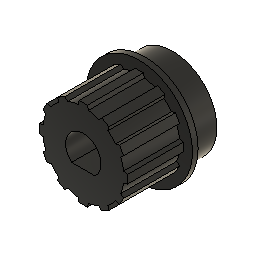
ENGRENAGEM_PEQUENA Modificada v1 (Autodesk Fusion 360 design; units mm, degrees)
Autodesk Fusion 360 part; units mm, degrees
sketch "Esboço1" plane through (0, 0, 0) normal (0, 1, 0) x (1, 0, 0)
  circle A0 centre (0, 0) radius 7.825
  line L0 (7.825, 0) -> (-7.825, 0) construction
  line L1 (0, 0) -> (0, -9.175) construction
  line L2 (0, 0) -> (0, 9.175) construction
  circle A1 centre (0, 0) radius 4
  circle A2 centre (0, 0) radius 9.175
  line L3 (-0.935, -9.9864) -> (0.935, -9.9864)
  line L4 (-1.55, -7.6699) -> (1.55, -7.6699)
  line L5 (-1.55, -7.6699) -> (-0.935, -9.9864)
  line L6 (0.935, -9.9864) -> (1.55, -7.6699)
  line L7 (4.1835, -9.116) -> (5.8029, -8.181)
  line L8 (2.4926, -7.4174) -> (5.1773, -5.8674)
  line L9 (2.4926, -7.4174) -> (4.1835, -9.116)
  line L10 (5.8029, -8.181) -> (5.1773, -5.8674)
  line L11 (8.181, -5.8029) -> (9.116, -4.1835)
  line L12 (5.8674, -5.1773) -> (7.4174, -2.4926)
  line L13 (5.8674, -5.1773) -> (8.181, -5.8029)
  line L14 (9.116, -4.1835) -> (7.4174, -2.4926)
  line L15 (9.9864, -0.935) -> (9.9864, 0.935)
  line L16 (7.6699, -1.55) -> (7.6699, 1.55)
  line L17 (7.6699, -1.55) -> (9.9864, -0.935)
  line L18 (9.9864, 0.935) -> (7.6699, 1.55)
  line L19 (9.116, 4.1835) -> (8.181, 5.8029)
  line L20 (7.4174, 2.4926) -> (5.8674, 5.1773)
  line L21 (7.4174, 2.4926) -> (9.116, 4.1835)
  line L22 (8.181, 5.8029) -> (5.8674, 5.1773)
  line L23 (5.8029, 8.181) -> (4.1835, 9.116)
  line L24 (5.1773, 5.8674) -> (2.4926, 7.4174)
  line L25 (5.1773, 5.8674) -> (5.8029, 8.181)
  line L26 (4.1835, 9.116) -> (2.4926, 7.4174)
  line L27 (0.935, 9.9864) -> (-0.935, 9.9864)
  line L28 (1.55, 7.6699) -> (-1.55, 7.6699)
  line L29 (1.55, 7.6699) -> (0.935, 9.9864)
  line L30 (-0.935, 9.9864) -> (-1.55, 7.6699)
  line L31 (-4.1835, 9.116) -> (-5.8029, 8.181)
  line L32 (-2.4926, 7.4174) -> (-5.1773, 5.8674)
  line L33 (-2.4926, 7.4174) -> (-4.1835, 9.116)
  line L34 (-5.8029, 8.181) -> (-5.1773, 5.8674)
  line L35 (-8.181, 5.8029) -> (-9.116, 4.1835)
  line L36 (-5.8674, 5.1773) -> (-7.4174, 2.4926)
  line L37 (-5.8674, 5.1773) -> (-8.181, 5.8029)
  line L38 (-9.116, 4.1835) -> (-7.4174, 2.4926)
  line L39 (-9.9864, 0.935) -> (-9.9864, -0.935)
  line L40 (-7.6699, 1.55) -> (-7.6699, -1.55)
  line L41 (-7.6699, 1.55) -> (-9.9864, 0.935)
  line L42 (-9.9864, -0.935) -> (-7.6699, -1.55)
  line L43 (-9.116, -4.1835) -> (-8.181, -5.8029)
  line L44 (-7.4174, -2.4926) -> (-5.8674, -5.1773)
  line L45 (-7.4174, -2.4926) -> (-9.116, -4.1835)
  line L46 (-8.181, -5.8029) -> (-5.8674, -5.1773)
  line L47 (-5.8029, -8.181) -> (-4.1835, -9.116)
  line L48 (-5.1773, -5.8674) -> (-2.4926, -7.4174)
  line L49 (-5.1773, -5.8674) -> (-5.8029, -8.181)
  line L50 (-4.1835, -9.116) -> (-2.4926, -7.4174)
  dimension "d1" = 15.65
  dimension "d3" = 9.175
  dimension "d4" = 9.175
  dimension "d10" = 8
  dimension "d33" = 18.35
  dimension "d42" = 1.87
  dimension "d43" = 3.1
  dimension "d47" = 1.55
  dimension "d48" = 0.935
  dimension "d50" = 360
  constraint coincident A0.centre L1.start
  constraint coincident A0 L0.start
  constraint coincident A0 L0.end
  constraint perpendicular L0 L1
  constraint perpendicular L0 L2
  constraint concentric A0 A2
  constraint perpendicular L1 L3
  constraint perpendicular L1 L4
  constraint coincident L1.end A2
  constraint vertical L1
  constraint coincident A0 L4.end
  measures "d1" diameter of A0
  measures "d3" distance of A0.centre L1.end
  measures "d4" distance of A0.centre L2.end
  measures "d10" diameter of A1
  measures "d33" diameter of A2
  measures "d42" distance of L3.start L3.end
  measures "d43" distance of L4.start L4.end
  measures "d47" distance of L1 L4.start
  measures "d48" distance of L1 L3.start
extrude "Extrusão1" add sketch "Esboço1" along normal blind 12.65 makes body 1
sketch "Esboço2" plane through (0, 12.65, 0) normal (0, 1, 0) x (-1, 0, 0)
  circle A0 centre (0, 0) radius 4
  circle A1 centre (0, 0) radius 12
  line L0 (4.1835, 9.116) -> (3.5365, 8.466)
  arc A2 (3.5365, 8.466) -> (1.1703, 9.1001) centre (0, 0) ccw
  line L1 (1.1703, 9.1001) -> (0.935, 9.9864)
  line L2 (0.935, 9.9864) -> (-0.935, 9.9864)
  line L3 (-0.935, 9.9864) -> (-1.1703, 9.1001)
  arc A3 (-1.1703, 9.1001) -> (-3.5365, 8.466) centre (0, 0) ccw
  line L4 (-3.5365, 8.466) -> (-4.1835, 9.116)
  line L5 (-4.1835, 9.116) -> (-5.8029, 8.181)
  line L6 (-5.8029, 8.181) -> (-5.5636, 7.2957)
  arc A4 (-5.5636, 7.2957) -> (-7.2957, 5.5636) centre (0, 0) ccw
  line L7 (-7.2957, 5.5636) -> (-8.181, 5.8029)
  line L8 (-8.181, 5.8029) -> (-9.116, 4.1835)
  line L9 (-9.116, 4.1835) -> (-8.466, 3.5365)
  arc A5 (-8.466, 3.5365) -> (-9.1001, 1.1703) centre (0, 0) ccw
  line L10 (-9.1001, 1.1703) -> (-9.9864, 0.935)
  line L11 (-9.9864, 0.935) -> (-9.9864, -0.935)
  line L12 (-9.9864, -0.935) -> (-9.1001, -1.1703)
  arc A6 (-9.1001, -1.1703) -> (-8.466, -3.5365) centre (0, 0) ccw
  line L13 (-8.466, -3.5365) -> (-9.116, -4.1835)
  line L14 (-9.116, -4.1835) -> (-8.181, -5.8029)
  line L15 (-8.181, -5.8029) -> (-7.2957, -5.5636)
  arc A7 (-7.2957, -5.5636) -> (-5.5636, -7.2957) centre (0, 0) ccw
  line L16 (-5.5636, -7.2957) -> (-5.8029, -8.181)
  line L17 (-5.8029, -8.181) -> (-4.1835, -9.116)
  line L18 (-4.1835, -9.116) -> (-3.5365, -8.466)
  arc A8 (-3.5365, -8.466) -> (-1.1703, -9.1001) centre (0, 0) ccw
  line L19 (-1.1703, -9.1001) -> (-0.935, -9.9864)
  line L20 (-0.935, -9.9864) -> (0.935, -9.9864)
  line L21 (0.935, -9.9864) -> (1.1703, -9.1001)
  arc A9 (1.1703, -9.1001) -> (3.5365, -8.466) centre (0, 0) ccw
  line L22 (3.5365, -8.466) -> (4.1835, -9.116)
  line L23 (4.1835, -9.116) -> (5.8029, -8.181)
  line L24 (5.8029, -8.181) -> (5.5636, -7.2957)
  arc A10 (5.5636, -7.2957) -> (7.2957, -5.5636) centre (0, 0) ccw
  line L25 (7.2957, -5.5636) -> (8.181, -5.8029)
  line L26 (8.181, -5.8029) -> (9.116, -4.1835)
  line L27 (9.116, -4.1835) -> (8.466, -3.5365)
  arc A11 (8.466, -3.5365) -> (9.1001, -1.1703) centre (0, 0) ccw
  line L28 (9.1001, -1.1703) -> (9.9864, -0.935)
  line L29 (9.9864, -0.935) -> (9.9864, 0.935)
  line L30 (9.9864, 0.935) -> (9.1001, 1.1703)
  arc A12 (9.1001, 1.1703) -> (8.466, 3.5365) centre (0, 0) ccw
  line L31 (8.466, 3.5365) -> (9.116, 4.1835)
  line L32 (9.116, 4.1835) -> (8.181, 5.8029)
  line L33 (8.181, 5.8029) -> (7.2957, 5.5636)
  arc A13 (7.2957, 5.5636) -> (5.5636, 7.2957) centre (0, 0) ccw
  line L34 (5.5636, 7.2957) -> (5.8029, 8.181)
  line L35 (5.8029, 8.181) -> (4.1835, 9.116)
  dimension "d13" = 24
  constraint coincident A0.centre A1.centre
  measures "d13" diameter of A1
extrude "Extrusão2" add sketch "Esboço2" along normal blind 1.3 separate body contours A1 | L0 A2 L1 L2 L3 A3 L4 L5 L6 A4 L7 L8 L9 A5 L10 L11 L12 A6 L13 L14 L15 A7 L16 L17 L18 A8 L19 L20 L21 A9 L22 L23 L24 A10 L25 L26 L27 A11 L28 L29 L30 A12 L31 L32 L33 A13 L34 L35 makes body 2
sketch "Esboço3" plane through (0, 13.95, 0) normal (0, 1, 0) x (-1, 0, 0)
  circle A0 centre (0, 0) radius 4
  circle A1 centre (0, 0) radius 12
  circle A2 centre (0, 0) radius 10
  dimension "d16" = 20
  constraint coincident A0.centre A1.centre
  measures "d16" diameter of A2
extrude "Extrusão3" add sketch "Esboço3" along normal blind 6.25 contours A2 bodies 2
sketch "Esboço4" plane through (0, 20.2, 0) normal (0, 1, 0) x (-1, 0, 0)
  circle A0 centre (0, 0) radius 4
  circle A1 centre (0, 0) radius 10
  circle A2 centre (0, 0) radius 6
  line L0 (0, 0) -> (0, -8.9799) construction
  line L1 (0, -5.9921) -> (-2.85, -5.9921)
  line L2 (-2.85, -5.9921) -> (-2.85, -7.9921)
  line L3 (-2.85, -7.9921) -> (0, -7.9921)
  line L4 (0, -5.9921) -> (2.85, -5.9921)
  line L5 (2.85, -5.9921) -> (2.85, -7.9921)
  line L6 (2.85, -7.9921) -> (0, -7.9921)
  line L7 (2.85, -5.9921) -> (2.85, -5.2799)
  line L8 (-2.85, -5.9921) -> (-2.85, -5.2799)
  dimension "d19" = 12
  dimension "d20" = 2.85
  dimension "d21" = 2.85
  dimension "d22" = 2
  constraint coincident A0.centre A1.centre
  constraint vertical L0
  constraint coincident L0 L1.start
  constraint perpendicular L0 L1
  constraint perpendicular L1 L2
  constraint coincident L0 L3.end
  constraint perpendicular L2 L3
  constraint perpendicular L0 L4
  constraint perpendicular L4 L5
  constraint perpendicular L0 L6
  constraint coincident A2 L7.end
  constraint perpendicular L4 L7
  constraint symmetric L0 L4.end L1.end
  constraint symmetric L0 L7.end L8.end
  measures "d19" diameter of A2
  measures "d20" distance of L3.end L5.end
  measures "d21" distance of L2.end L3.end
  measures "d22" distance of L4.end L5.end
extrude "Extrusão4" cut sketch "Esboço4" against normal blind 6 contours A2 L1 L8 | A2 L4 L7 | A2 L1 L2 L3 L4 L5 L6 bodies 2
sketch "Esboço5" plane through (0, 0, -7.9921) normal (0, 0, 1) x (-1, 0, 0)
  line L0 (-2.85, -20.2) -> (2.85, -20.2)
  line L1 (2.85, -20.2) -> (2.85, -14.2)
  line L2 (2.85, -14.2) -> (-2.85, -14.2)
  line L3 (-2.85, -14.2) -> (-2.85, -20.2)
  circle A0 centre (0, -17) radius 1.65
  dimension "d25" = 3.3
  measures "d25" diameter of A0
extrude "Extrusão5" cut sketch "Esboço5" along normal blind 5 and the other way blind 2.008 contours A0 bodies 2
sketch "Esboço6" plane through (0, 0, 0) normal (0, -1, 0) x (1, 0, 0)
  circle A0 centre (0, 0) radius 4
  line L0 (0, -4) -> (0, -3) construction
  line L1 (0, -3) -> (-2.6458, -3)
  line L2 (0, -3) -> (2.6458, -3)
  line L3 (-3.5365, 8.466) -> (-4.1835, 9.116)
  line L4 (-4.1835, 9.116) -> (-5.8029, 8.181)
  line L5 (-5.8029, 8.181) -> (-5.5636, 7.2957)
  arc A1 (-5.5636, 7.2957) -> (-7.2957, 5.5636) centre (0, 0) ccw
  line L6 (-7.2957, 5.5636) -> (-8.181, 5.8029)
  line L7 (-8.181, 5.8029) -> (-9.116, 4.1835)
  line L8 (-9.116, 4.1835) -> (-8.466, 3.5365)
  arc A2 (-8.466, 3.5365) -> (-9.1001, 1.1703) centre (0, 0) ccw
  line L9 (-9.1001, 1.1703) -> (-9.9864, 0.935)
  line L10 (-9.9864, 0.935) -> (-9.9864, -0.935)
  line L11 (-9.9864, -0.935) -> (-9.1001, -1.1703)
  arc A3 (-9.1001, -1.1703) -> (-8.466, -3.5365) centre (0, 0) ccw
  line L12 (-8.466, -3.5365) -> (-9.116, -4.1835)
  line L13 (-9.116, -4.1835) -> (-8.181, -5.8029)
  line L14 (-8.181, -5.8029) -> (-7.2957, -5.5636)
  arc A4 (-7.2957, -5.5636) -> (-5.5636, -7.2957) centre (0, 0) ccw
  line L15 (-5.5636, -7.2957) -> (-5.8029, -8.181)
  line L16 (-5.8029, -8.181) -> (-4.1835, -9.116)
  line L17 (-4.1835, -9.116) -> (-3.5365, -8.466)
  arc A5 (-3.5365, -8.466) -> (-1.1703, -9.1001) centre (0, 0) ccw
  line L18 (-1.1703, -9.1001) -> (-0.935, -9.9864)
  line L19 (-0.935, -9.9864) -> (0.935, -9.9864)
  line L20 (0.935, -9.9864) -> (1.1703, -9.1001)
  arc A6 (1.1703, -9.1001) -> (3.5365, -8.466) centre (0, 0) ccw
  line L21 (3.5365, -8.466) -> (4.1835, -9.116)
  line L22 (4.1835, -9.116) -> (5.8029, -8.181)
  line L23 (5.8029, -8.181) -> (5.5636, -7.2957)
  arc A7 (5.5636, -7.2957) -> (7.2957, -5.5636) centre (0, 0) ccw
  line L24 (7.2957, -5.5636) -> (8.181, -5.8029)
  line L25 (8.181, -5.8029) -> (9.116, -4.1835)
  line L26 (9.116, -4.1835) -> (8.466, -3.5365)
  arc A8 (8.466, -3.5365) -> (9.1001, -1.1703) centre (0, 0) ccw
  line L27 (9.1001, -1.1703) -> (9.9864, -0.935)
  line L28 (9.9864, -0.935) -> (9.9864, 0.935)
  line L29 (9.9864, 0.935) -> (9.1001, 1.1703)
  arc A9 (9.1001, 1.1703) -> (8.466, 3.5365) centre (0, 0) ccw
  line L30 (8.466, 3.5365) -> (9.116, 4.1835)
  line L31 (9.116, 4.1835) -> (8.181, 5.8029)
  line L32 (8.181, 5.8029) -> (7.2957, 5.5636)
  arc A10 (7.2957, 5.5636) -> (5.5636, 7.2957) centre (0, 0) ccw
  line L33 (5.5636, 7.2957) -> (5.8029, 8.181)
  line L34 (5.8029, 8.181) -> (4.1835, 9.116)
  line L35 (4.1835, 9.116) -> (3.5365, 8.466)
  arc A11 (3.5365, 8.466) -> (1.1703, 9.1001) centre (0, 0) ccw
  line L36 (1.1703, 9.1001) -> (0.935, 9.9864)
  line L37 (0.935, 9.9864) -> (-0.935, 9.9864)
  line L38 (-0.935, 9.9864) -> (-1.1703, 9.1001)
  arc A12 (-1.1703, 9.1001) -> (-3.5365, 8.466) centre (0, 0) ccw
  constraint coincident A0 L0.start
  constraint vertical L0
  constraint coincident A0 L1.end
  constraint perpendicular L0 L1
  constraint coincident A0 L2.end
  constraint perpendicular L0 L2
extrude "Extrusão6" add sketch "Esboço6" against normal blind 10 contours A0 L1 L2 picked at (-0.1921, -3.6528) bodies 1
